script OS 4_v1 (Autodesk Fusion 360 design; units mm, degrees)
Autodesk Fusion 360 part; units mm, degrees
sketch "right content" plane through (0, 0, 0) normal (0, 0, 1) x (1, 0, 0)
  line L0 (-306, -8) -> (-256, -8) construction
  line L1 (-256, -128) -> (-306, -128) construction
  line L2 (-256, -8) -> (-256, -128) construction
  line L3 (-306, -128) -> (-306, -8) construction
  circle A0 centre (-298, -98) radius 1.005 construction
  point P0 (-294, -98)
  point P1 (-290, -98)
  point P2 (-298, -94)
  point P3 (-294, -94)
  point P4 (-290, -94)
  point P5 (-298, -90)
  point P6 (-294, -90)
  point P7 (-290, -90)
  point P8 (-298, -86)
  point P9 (-294, -86)
  point P10 (-290, -86)
  point P11 (-298, -82)
  point P12 (-294, -82)
  point P13 (-290, -82)
  point P14 (-298, -78)
  point P15 (-294, -78)
  point P16 (-290, -78)
  point P17 (-298, -74)
  point P18 (-294, -74)
  point P19 (-290, -74)
  point P20 (-298, -70)
  point P21 (-294, -70)
  point P22 (-290, -70)
  point P23 (-298, -66)
  point P24 (-294, -66)
  point P25 (-290, -66)
  point P26 (-298, -62)
  point P27 (-294, -62)
  point P28 (-290, -62)
  dimension "d85" = 50
  dimension "d390" = 120
  dimension "d391" = 2.01
  dimension "d394" = 4
  dimension "d395" = 4
  dimension "d403" = 30
  dimension "d404" = 8
  constraint horizontal L1
  constraint horizontal L0
  constraint vertical L2
  constraint vertical L3
  constraint coincident L1.end L3.start
  constraint coincident L0.end L2.start
  measures "d85" distance of L0.start L0.end
  measures "d390" distance of L0 L1
  measures "d391" diameter of A0
  measures "d403" distance of L1 A0.centre
  measures "d404" distance of L3 A0.centre
sketch "top content" plane through (0, 0, 0) normal (0, 0, 1) x (1, 0, 0)
  circle A0 centre (-155, -115.7409) radius 6.5
  circle A1 centre (-223, -61) radius 6.5
  circle A2 centre (-139.5, -131.2409) radius 1.588
  line L0 (-128.7151, -190.6415) -> (-249.2849, -41.0991) construction
  circle A3 centre (-189, -115.8703) radius 1.588
  line L1 (-128.7151, -190.6415) -> (-248.7143, -191.098) construction
  line L2 (-129.2857, -40.6426) -> (-128.7151, -190.6415) construction
  line L3 (-129.2857, -40.6426) -> (-248.7143, -191.098) construction
  circle A4 centre (-170.5, -131.2409) radius 1.588
  circle A5 centre (-139.5, -100.2409) radius 1.588
  line L4 (-248.7143, -191.098) -> (-249.2849, -41.0991) construction
  circle A6 centre (-170.5, -100.2409) radius 1.588
  line L5 (-249.2849, -41.0991) -> (-129.2857, -40.6426) construction
  circle A7 centre (-223, -171) radius 6.5
  point P0 (-189, -115.8703)
  point P1 (-189, -115.8703)
  dimension "d263" = 31
  dimension "d25" = 31
  dimension "d1" = 150
  dimension "d2" = 120
  dimension "d3" = 13
  dimension "d4" = 110
  dimension "d272" = 3.176
  dimension "d408" = 75
  dimension "d1144" = 34
  dimension "d1145" = 15.5
  dimension "d1146" = 15.5
  dimension "d1147" = 20
  dimension "d1148" = 34
  dimension "d1149" = 25.9998
  constraint perpendicular L1 L2
  constraint parallel L2 L4
  constraint parallel L1 L5
  constraint coincident P1 L3
  constraint coincident P1 L0
  constraint coincident P1 P0
  constraint equal A0 A1
  constraint equal A1 A7
  constraint vertical A7.centre A1.centre
  measures "d1" distance of L0.start L2.start
  measures "d2" distance of L0.end L2.start
  measures "d3" diameter of A1
  measures "d4" distance of A7.centre A1.centre
  measures "d272" diameter of A4
  measures "d408" distance of A0.centre L1
  measures "d1144" horizontal distance of A1.centre P1
  measures "d1145" horizontal distance of A0.centre A4.centre
  measures "d1146" vertical distance of A0.centre A4.centre
  measures "d1147" distance of A7.centre L1
  measures "d1148" horizontal distance of A0.centre P0
  measures "d1149" distance of A0.centre L2
sketch "bottom content" plane through (0, 0, 0) normal (0, 0, 1) x (1, 0, 0)
  circle A0 centre (245.4709, 45.6033) radius 1
  circle A1 centre (385.4709, 45.6033) radius 1
  circle A2 centre (245.4709, -54.3967) radius 1
  circle A3 centre (385.4709, -54.3967) radius 1
  circle A4 centre (255.4709, 35.6033) radius 1
  circle A5 centre (375.4709, 35.6033) radius 1
  circle A6 centre (255.4709, -44.3967) radius 1
  circle A7 centre (375.4709, -44.3967) radius 1
  line L0 (235.4709, 55.6033) -> (395.4709, 55.6033) construction
  line L1 (395.4709, 55.6033) -> (395.4709, -64.3967) construction
  line L2 (395.4709, -64.3967) -> (235.4709, -64.3967) construction
  line L3 (235.4709, -64.3967) -> (235.4709, 55.6033) construction
  line L4 (235.4709, 55.6033) -> (395.4709, -64.3967) construction
  line L5 (395.4709, 55.6033) -> (235.4709, -64.3967) construction
  line L6 (268.4709, -6.3967) -> (362.4709, -6.3967) construction
  line L7 (362.4709, -6.3967) -> (362.4709, -54.3967) construction
  line L8 (362.4709, -54.3967) -> (268.4709, -54.3967) construction
  line L9 (268.4709, -54.3967) -> (268.4709, -6.3967) construction
  line L10 (315.4709, -4.3967) -> (315.4709, -64.3967) construction
  circle A8 centre (268.4709, -6.3967) radius 1
  circle A9 centre (362.4709, -6.3967) radius 1
  circle A10 centre (362.4709, -54.3967) radius 1
  circle A11 centre (268.4709, -54.3967) radius 1
  point P0 (315.4709, -4.3967)
  point P1 (315.4709, -4.3967)
  dimension "d282" = 2
  dimension "d287" = 140
  dimension "d288" = -100
  dimension "d289" = 2
  dimension "d294" = 120
  dimension "d295" = -80
  dimension "d356" = 160
  dimension "d357" = 120
  dimension "d358" = 70
  dimension "d359" = 50
  dimension "d360" = 60
  dimension "d361" = 40
  dimension "d362" = 94
  dimension "d363" = 48
  dimension "d364" = 10
  dimension "d365" = 47
  dimension "d366" = 2
  dimension "d368" = 2
  dimension "d369" = 2
  dimension "d370" = 2
  constraint horizontal L0
  constraint perpendicular L0 L1
  constraint parallel L0 L2
  constraint parallel L1 L3
  constraint coincident L4 P1
  constraint coincident L5 P1
  constraint coincident P1 P0
  constraint horizontal L6
  constraint vertical L7
  constraint horizontal L8
  constraint vertical L9
  constraint midpoint L2 L10.end
  constraint coincident L6.start L9.end
  constraint coincident L6.end L7.start
  constraint coincident L7.end L8.start
  constraint coincident L8.end L9.start
  measures "d282" diameter of A0
  measures "d289" diameter of A4
  measures "d356" distance of L1.end L2.end
  measures "d357" distance of L0.start L2.end
  measures "d358" horizontal distance of A0.centre P0
  measures "d359" vertical distance of A0.centre P0
  measures "d360" horizontal distance of A4.centre P1
  measures "d361" vertical distance of A4.centre P1
  measures "d362" distance of L6.start L6.end
  measures "d363" distance of L6.start L8.end
  measures "d364" distance of L2 L8
  measures "d365" distance of L8.end L10
  measures "d366" diameter of A8
  measures "d368" diameter of A11
  measures "d369" diameter of A9
  measures "d370" diameter of A10
sketch "back content" plane through (0, 0, 0) normal (0, 0, 1) x (1, 0, 0)
  line L0 (16.9082, 180.3872) -> (176.9082, 180.3872) construction
  line L1 (176.9082, 180.3872) -> (176.9082, 130.3872) construction
  line L2 (176.9082, 130.3872) -> (16.9082, 130.3872) construction
  line L3 (16.9082, 130.3872) -> (16.9082, 180.3872) construction
  circle A0 centre (156.9082, 150.3872) radius 5.6
  dimension "d381" = 160
  dimension "d382" = 50
  dimension "d387" = 11.2
  dimension "d388" = 20
  dimension "d389" = 20
  constraint horizontal L0
  constraint horizontal L2
  constraint vertical L3
  constraint vertical L1
  measures "d381" distance of L0.start L0.end
  measures "d382" distance of L0.start L2.end
  measures "d387" diameter of A0
  measures "d388" distance of L2 A0.centre
  measures "d389" distance of L1 A0.centre
sketch "front content" plane through (0, 0, 0) normal (0, 0, 1) x (1, 0, 0)
  line L0 (-253.343, 200.8306) -> (-230.343, 200.8306)
  line L1 (-230.343, 200.8306) -> (-230.343, 190.3306)
  line L2 (-230.343, 190.3306) -> (-253.343, 190.3306)
  line L3 (-253.343, 190.3306) -> (-253.343, 200.8306)
  circle A0 centre (-183.343, 190.8306) radius 3.5
  line L4 (-143.343, 185.8306) -> (-128.343, 185.8306)
  line L5 (-128.343, 185.8306) -> (-128.343, 177.8306)
  line L6 (-128.343, 177.8306) -> (-143.343, 177.8306)
  line L7 (-143.343, 177.8306) -> (-143.343, 185.8306)
  line L8 (-273.343, 215.8306) -> (-113.343, 215.8306) construction
  line L9 (-113.343, 215.8306) -> (-113.343, 165.8306) construction
  line L10 (-113.343, 165.8306) -> (-273.343, 165.8306) construction
  line L11 (-273.343, 165.8306) -> (-273.343, 215.8306) construction
  dimension "d332" = 23
  dimension "d333" = 10.5
  dimension "d336" = 7
  dimension "d339" = 15
  dimension "d340" = 8
  dimension "d371" = 160
  dimension "d372" = 50
  dimension "d374" = 20
  dimension "d376" = 15
  dimension "d377" = 12
  dimension "d378" = 15
  dimension "d379" = 25
  dimension "d380" = 70
  constraint horizontal L0
  constraint vertical L1
  constraint horizontal L2
  constraint vertical L3
  constraint horizontal L4
  constraint vertical L5
  constraint horizontal L6
  constraint vertical L7
  constraint horizontal L8
  constraint vertical L9
  constraint horizontal L10
  constraint vertical L11
  measures "d332" distance of L0.start L0.end
  measures "d333" distance of L0.start L2.end
  measures "d336" diameter of A0
  measures "d339" distance of L4.start L4.end
  measures "d340" distance of L4.start L6.end
  measures "d371" distance of L8.start L8.end
  measures "d372" distance of L8.start L10.end
  measures "d374" distance of L3 L11
  measures "d376" distance of L0 L8
  measures "d377" distance of L6 L10
  measures "d378" distance of L5 L9
  measures "d379" distance of A0.centre L10
  measures "d380" distance of A0.centre L9
sketch "left content" plane through (0, 0, 0) normal (0, 0, 1) x (1, 0, 0)
  line L0 (131.529, -3.2484) -> (131.529, 116.7516) construction
  circle A0 centre (139.529, 26.7516) radius 1.005 construction
  line L1 (181.529, -3.2484) -> (131.529, -3.2484) construction
  line L2 (131.529, 116.7516) -> (181.529, 116.7516) construction
  line L3 (181.529, 116.7516) -> (181.529, -3.2484) construction
  point P0 (139.529, 34.7516)
  point P1 (147.529, 50.7516)
  point P2 (139.529, 54.7516)
  point P3 (143.529, 54.7516)
  point P4 (147.529, 34.7516)
  point P5 (139.529, 30.7516)
  point P6 (143.529, 30.7516)
  point P7 (143.529, 50.7516)
  point P8 (143.529, 34.7516)
  point P9 (139.529, 38.7516)
  point P10 (147.529, 38.7516)
  point P11 (139.529, 42.7516)
  point P12 (143.529, 38.7516)
  point P13 (139.529, 46.7516)
  point P14 (147.529, 42.7516)
  point P15 (143.529, 46.7516)
  point P16 (147.529, 46.7516)
  point P17 (139.529, 50.7516)
  point P18 (143.529, 42.7516)
  point P19 (147.529, 30.7516)
  point P20 (147.529, 26.7516)
  point P21 (143.529, 26.7516)
  point P22 (143.529, 58.7516)
  point P23 (143.529, 62.7516)
  point P24 (147.529, 54.7516)
  point P25 (139.529, 58.7516)
  point P26 (147.529, 58.7516)
  point P27 (139.529, 62.7516)
  point P28 (147.529, 62.7516)
  dimension "d398" = 4
  dimension "d399" = 4
  dimension "d400" = 50
  dimension "d401" = 120
  dimension "d402" = 2.01
  dimension "d405" = 30
  dimension "d406" = 8
  constraint horizontal L1
  constraint horizontal L2
  constraint vertical L3
  constraint vertical L0
  constraint coincident L0.start L1.end
  constraint coincident L2.end L3.start
  measures "d400" distance of L2.end L0.end
  measures "d401" distance of L1 L2
  measures "d402" diameter of A0
  measures "d405" distance of A0.centre L1
  measures "d406" distance of A0.centre L0
sketch "b  stock" plane through (0, 0, 0) normal (0, 0, 1) x (1, 0, 0)
  line L0 (0, 0) -> (304.8, 0)
  line L1 (304.8, 0) -> (304.8, 609.6)
  line L2 (304.8, 609.6) -> (0, 609.6)
  line L3 (0, 609.6) -> (0, 0)
extrude "b  stock body extrude" add sketch "b  stock" along normal blind 3.175
sketch "imported OS" plane through (0, 0, 0) normal (0, 0, 1) x (1, 0, 0)
  circle A0 centre (207.5547, -0.7227) radius 12
  circle A1 centre (254.2547, 40.2773) radius 12
  line L0 (181.5547, 98.2773) -> (277.5547, 98.2773)
  line L1 (277.5547, 98.2773) -> (277.5547, -17.7227)
  line L2 (277.5547, -17.7227) -> (181.5547, -17.7227)
  line L3 (181.5547, -17.7227) -> (181.5547, 98.2773)
  line L4 (181.5547, 98.2773) -> (277.5547, -17.7227) construction
  line L5 (277.5547, 98.2773) -> (181.5547, -17.7227) construction
  line L6 (181.5547, 40.2773) -> (277.5547, 40.2773) construction
  circle A2 centre (207.5547, 81.2773) radius 12
  point P0 (229.5547, 40.2773)
  dimension "d1359" = 24
  dimension "d1361" = 24
  dimension "d1362" = 96
  dimension "d1363" = 116
  dimension "d1364" = 26
  dimension "d1365" = 17
  dimension "d1366" = 46.7
  constraint perpendicular L0 L1
  constraint parallel L1 L3
  constraint coincident L4 P0
  constraint coincident L5 P0
  constraint midpoint L3 L6.start
  constraint midpoint L1 L6.end
  constraint symmetric A0 L6 A2
  constraint coincident A1.centre L6
  constraint horizontal L2
  constraint vertical L1
  measures "d1359" diameter of A0
  measures "d1361" diameter of A1
  measures "d1362" distance of L1.end L2.end
  measures "d1363" distance of L0.end L1.end
  measures "d1364" distance of A0.centre L3
  measures "d1365" distance of A0.centre L2
  measures "d1366" horizontal distance of A0.centre A1.centre
equation "toolDiameter = 2.01 mm"
equation "d272 = screwHoleSize"
equation "d282 = pcbMountHoles"
equation "d289 = pcbMountHoles"
equation "screwHoleSize = 3.176 mm"
equation "d366 = pcbMountHoles"
equation "pcbMountHoles = 2 mm"
equation "d368 = pcbMountHoles"
equation "d369 = pcbMountHoles"
equation "d370 = pcbMountHoles"
equation "d391 = toolDiameter"
equation "d402 = toolDiameter"
equation "Length = 150.0 mm" comment "Length (mm)"
equation "Depth = 120.0 mm" comment "Depth (mm)"
equation "Height = 50.0 mm" comment "Height (mm)"
equation "Thickness = 3.175 mm" comment "Thickness (mm)"
equation "Tool_diameter = 2.01 mm" comment "Tool Diameter (mm)"
equation "Tooth_width = 10.0 mm" comment "Target Tooth Width (mm)"
equation "Kerf = -0.1 mm" comment "Kerf (mm)- can be negative"
equation "Delta_from_bottom = -0.1 mm" comment "Additional fine adjustment of bone centers from bottom of holes(mm)- positive makes smaller bottom indents"
equation "Stock_x_dimension = 304.8 mm" comment "Stock X Dimension"
equation "Stock_y_dimension = 609.6 mm" comment "Stock Y Dimension"
equation "Repeats_l_tmp = -1.0 mm" comment "temp hidden"
named bodies: "b  stock body"
